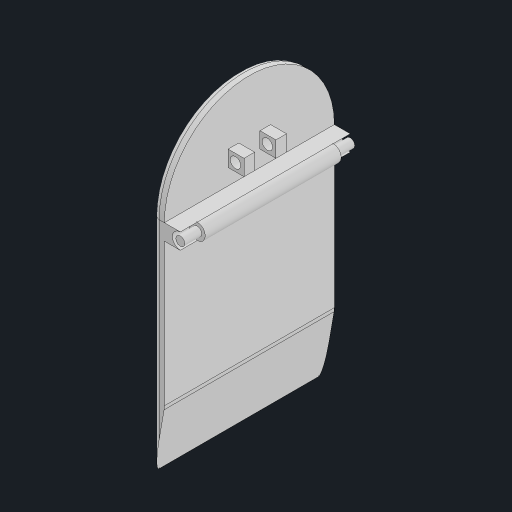
# Autodesk Inventor part: 집게 이동
Saved by Autodesk Inventor 2024.1 (Build 281209000, 209)
## iProperties
Created: 2024-01-27
Part Number: 집게 이동
Material: 일반
Document SubType Name: Modeling
Designer: likek
Density: 1 g/cm^3
Appearance: 기본값
Author: likek
Autodesk Inventor part; units mm, degrees
ref_plane "YZ Plane" through (0, 0, 0) normal (1, 0, 0) x (0, 1, 0)
ref_plane "XZ Plane" through (0, 0, 0) normal (0, 1, 0) x (-1, 0, 0)
ref_plane "XY Plane" through (0, 0, 0) normal (0, 0, 1) x (1, 0, 0)
sketch "스케치1" plane through (0, 0, 0) normal (0, 0, 1) x (1, 0, 0)
  circle A0 centre (0, 0) radius 0.425
  circle A1 centre (0, 0) radius 0.75
  line L0 (0, 0.75) -> (-1.5, 0.75)
  line L1 (-1.5, 0.75) -> (-1.5, -0.75)
  line L2 (-1.5, -0.75) -> (0, -0.75)
  circle A2 centre (0, 0) radius 0.8
  point P0 (-0.2784, -0.75)
  point P1 (-0.2784, 0.75)
  dimension "d0" = 0.85
  dimension "d3" = 1.5
  dimension "d6" = 1.5
  dimension "d7" = 1.5
  dimension "d10" = 1.6
  constraints: 6 end point, 3 centre point, 3 coincident, 2 perpendicular, 2 point on circle, 1 horizontal
  measures "d0" diameter of A0
  measures "d3" diameter of A1
  measures "d6" distance of L0.start L0.end
  measures "d7" distance of L0.end L1.end
  measures "d10" diameter of A2
extrude "돌출1" add sketch "스케치1" along normal mid plane 16 contours A0
extrude "돌출2" add sketch "스케치1" along normal mid plane 12.8 contours A1
extrude "돌출3" add sketch "스케치1" along normal mid plane 16 contours A1 L2 A2 L0 | A2 L2 L1 L0 picked at (-0.763, 0)
extrude "돌출4" add sketch "스케치1" along normal mid plane 8 contours A2 L2 L1 L0
sketch "스케치2" plane through (-1.5, -0.75, 4) normal (-1, 0, 0) x (0, 0, 1)
  line L0 (4, 1.5) -> (4, 0)
  line L1 (-12, 1.5) -> (4, 1.5) projected
  line L2 (-12, 0) -> (-12, 1.5)
  arc A0 (4, 1.5) -> (-12, 1.5) centre (-4, 1.5) ccw
  line L3 (-12, 1.5) -> (-12, -20.5)
  line L4 (-12, -20.5) -> (4, -20.5)
  line L5 (4, -20.5) -> (4, 1.5)
  point P0 (-4, 0.75)
  dimension "d15" = 22
  dimension "d52" = 8
  dimension "d53" = 16
  dimension "d54" = 8
  constraints: 10 end point, 3 point on circle, 2 point on line, 1 centre point, 1 midpoint, 1 perpendicular, 1 vertical
  measures "d15" distance of L2.end L3.end
  measures "d52" radius of A0
  measures "d53" distance of L3.end L4.end
  measures "d54" distance from line of point (-4, 0.75) L3
extrude "돌출5" add sketch "스케치2" along normal blind 1
sketch "스케치4" plane through (-1.5, -0.75, 4) normal (1, 0, 0) x (0, 0, -1)
  line L0 (3.25, 3) -> (4.75, 3)
  line L1 (4.75, 3) -> (4.75, 4.5)
  line L2 (4.75, 4.5) -> (3.25, 4.5)
  line L3 (3.25, 4.5) -> (3.25, 3)
  line L4 (3.25, 3) -> (4.75, 4.5) construction
  line L5 (4.75, 3) -> (3.25, 4.5) construction
  line L6 (2, 3) -> (3, 3)
  line L7 (3, 3) -> (3, 4.5)
  line L8 (3, 4.5) -> (2, 4.5)
  line L9 (2, 4.5) -> (2, 3)
  line L10 (2, 3) -> (3, 4.5) construction
  line L11 (3, 3) -> (2, 4.5) construction
  line L12 (6, 3) -> (5, 3)
  line L13 (5, 3) -> (5, 4.5)
  line L14 (5, 4.5) -> (6, 4.5)
  line L15 (6, 4.5) -> (6, 3)
  line L16 (6, 3) -> (5, 4.5) construction
  line L17 (5, 3) -> (6, 4.5) construction
  point P0 (4, 0.75)
  point P1 (4, 3.75)
  point P2 (2.5, 3.75)
  point P3 (5.5, 3.75)
  dimension "d26" = 1.5
  dimension "d27" = 1.5
  dimension "d28" = 1
  dimension "d29" = 1
  dimension "d30" = 1.5
  dimension "d31" = 3
  dimension "d32" = 3
  constraints: 36 end point, 6 midpoint, 6 parallel, 3 horizontal, 3 perpendicular, 1 point on line, 1 vertical alignment
  measures "d26" distance of L0.end L1.end
  measures "d27" distance of L1.end L2.end
  measures "d28" distance of L7.end L8.end
  measures "d29" distance of L13.end L14.end
  measures "d30" distance of point (4, 3.75) point (2.5, 3.75)
  measures "d31" distance of point (2.5, 3.75) point (5.5, 3.75)
  measures "d32" distance of point (4, 0.75) point (4, 3.75)
extrude "돌출7" add sketch "스케치4" along normal blind 1.5 contours L9 L8 L7 L6 | L12 L13 L14 L15
sketch "스케치5" plane through (0, 0, 0) normal (0, 0, 1) x (1, 0, 0)
  circle A0 centre (-0.8043, 3) radius 0.5
  circle A1 centre (-0.8043, 3) radius 0.4
  line L0 (-0.8043, 2.5) -> (2.1886, 2.4792)
  line L1 (2.1886, 2.4792) -> (2.1957, 3.5)
  line L2 (2.1957, 3.5) -> (-0.8043, 3.5)
  point P0 (0, 0)
  dimension "d35" = 3
  dimension "d36" = 1
  dimension "d37" = 0.8
  dimension "d49" = 3
  constraints: 6 end point, 2 centre point, 2 point on circle, 1 coincident, 1 horizontal, 1 perpendicular
  measures "d35" vertical distance of point (0, 0) A0.centre
  measures "d36" diameter of A0
  measures "d37" diameter of A1
  measures "d49" distance of L1.end L2.end
extrude "돌출8" cut sketch "스케치5" along normal through all both and the other way through all contours A0 | A1
extrude "돌출9" [suppressed]
extrude "돌출10" [suppressed]
sketch "스케치6" plane through (0, 0, 8) normal (0, 0, 1) x (1, 0, 0)
  line L0 (-2.5, -21.25) -> (-2.5, 0.75) projected
  line L1 (-1.5, -21.25) -> (-2.5, -21.25) projected
  line L2 (-1.5, -21.25) -> (-1.5, -0.75) projected
  line L3 (-2.5, -20.055) -> (-1.5, -14.35)
  dimension "d55" = 1.195
  dimension "d61" = 6.9
  constraints: 2 end point, 2 point on line
  measures "d55" distance of L0.start L3.start
  measures "d61" distance of L1.start L3.end
extrude "돌출11" cut sketch "스케치6" against normal through all
fillet "모깎기9" radius 0.5 3 edges at (-2.5, 8.75, 0) (-2.5, -9.6525, -8) (-2.5, -9.6525, 8)
fillet "모깎기10" radius 2 1 edges at (-1.5, -14.35, 0)
equation "\"d29\" = d28"
